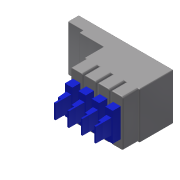
# Autodesk Inventor part: cRio FRC II with 3 modules 2 breakouts
Saved by Autodesk Inventor 2013 (Build 170138000, 138)
## iProperties
Created: 2013-12-22
Part Number: cRio FRC II with 3 modules 2 breakouts
Material: Iron, Cast
Document SubType Name: Modeling
Designer: Nemo
Mass: 1124.91 g
Surface Area: 772.846 cm^2
Volume: 929.109 cm^3
Density: 1.21074 g/cm^3
Author: Nemo
Autodesk Inventor part; units mm, degrees
ref_plane "YZ Plane" through (0, 0, 0) normal (1, 0, 0) x (0, 1, 0)
ref_plane "XZ Plane" through (0, 0, 0) normal (0, 1, 0) x (-1, 0, 0)
ref_plane "XY Plane" through (0, 0, 0) normal (0, 0, 1) x (1, 0, 0)
sketch "Sketch1" plane through (0, 0, 0) normal (0, 0, 1) x (1, 0, 0)
  line L0 (0, 0) -> (179.578, 0)
  line L1 (179.578, 0) -> (179.578, 88.138)
  line L2 (179.578, 88.138) -> (0, 88.138)
  line L3 (0, 88.138) -> (0, 0)
  dimension "d0" = 179.578
  dimension "d1" = 88.138
  constraints: 8 end point, 2 parallel, 1 horizontal, 1 perpendicular
  measures "d0" distance of L2.end L1.end
  measures "d1" distance of L1.end L0.end
extrude "Extrusion1" add sketch "Sketch1" along normal blind 27.94
sketch "Sketch2" plane through (0, 0, 27.94) normal (0, 0, 1) x (1, 0, 0)
  line L0 (0, 0) -> (179.578, 0) projected
  line L1 (179.578, 88.138) -> (75.184, 88.138)
  line L2 (75.184, 88.138) -> (75.184, 0)
  line L3 (75.184, 0) -> (179.578, 0)
  line L4 (179.578, 0) -> (179.578, 88.138)
  dimension "d4" = 104.394
  constraints: 8 end point, 2 parallel, 1 horizontal, 1 perpendicular, 1 point on line
  measures "d4" distance between parallel lines of L4 L2
extrude "Extrusion2" add sketch "Sketch2" along normal blind 36.3474
sketch "Sketch3" plane through (0, 0, 64.2874) normal (0, 0, 1) x (1, 0, 0)
  line L0 (75.184, 0) -> (179.578, 0) projected
  line L1 (179.578, 88.138) -> (75.184, 88.138) projected
  line L2 (75.184, 88.138) -> (75.184, 0) projected
  line L3 (77.724, 88.138) -> (100.584, 88.138)
  line L4 (100.584, 88.138) -> (100.584, 0)
  line L5 (100.584, 0) -> (77.724, 0)
  line L6 (77.724, 0) -> (77.724, 88.138)
  point P0 (0, 0)
  dimension "d8" = 22.86
  dimension "d9" = 2.54
  constraints: 8 end point, 2 parallel, 2 point on line, 1 horizontal, 1 perpendicular
  measures "d8" distance of L4.end L5.end
  measures "d9" distance between parallel lines of L2 L6
extrude "Extrusion3" add sketch "Sketch3" along normal blind 28.6512 contours L6 L1 L4 L0
fillet "Fillet1" radius 3.175 4 edges at (77.724, 0, 78.613) (100.584, 0, 78.613) (77.724, 88.138, 78.613) (100.584, 88.138, 78.613)
pattern_linear "Rectangular Pattern1" count 4 spacing 25.4 along (1, 0, 0) of "Extrusion3", "Fillet1"
sketch "Sketch4" plane through (0, 0, 27.94) normal (0, 0, 1) x (1, 0, 0)
  line L0 (75.184, 88.138) -> (0, 88.138) projected
  line L1 (0, 0) -> (28.956, 0)
  line L2 (28.956, 0) -> (28.956, 88.138)
  line L3 (28.956, 88.138) -> (0, 88.138)
  line L4 (0, 88.138) -> (0, 0)
  dimension "d16" = 28.956
  constraints: 8 end point, 2 parallel, 1 horizontal, 1 perpendicular, 1 point on line
  measures "d16" distance between parallel lines of L4 L2
extrude "Extrusion4" cut sketch "Sketch4" against normal blind 7.4422
fillet "Fillet2" radius 1.5875 64 edges at (28.956, 44.069, 27.94) (52.07, 0, 27.94) (75.184, 44.069, 27.94) (52.07, 88.138, 27.94) (14.478, 0, 20.4978) (0, 0, 10.2489) (89.789, 0, 0) (179.578, 0, 32.1437) (176.5935, 0, 64.2874) (165.354, 0, 92.9386) (152.654, 0, 64.2874) (139.954, 0, 92.9386) (127.254, 0, 64.2874) (114.554, 0, 92.9386) (101.854, 0, 64.2874) (89.154, 0, 92.9386) (78.0415, 0, 64.2874) (75.184, 0, 46.1137) (28.956, 0, 24.2189) (175.8541, 0.9299, 92.9386) (176.784, 44.069, 92.9386) (175.8541, 87.2081, 92.9386) (165.354, 88.138, 92.9386) (154.8539, 87.2081, 92.9386) (153.924, 44.069, 92.9386) (154.8539, 0.9299, 92.9386) (150.4541, 0.9299, 92.9386) (151.384, 44.069, 92.9386) (150.4541, 87.2081, 92.9386) (139.954, 88.138, 92.9386) (129.4539, 87.2081, 92.9386) (128.524, 44.069, 92.9386) (129.4539, 0.9299, 92.9386) (125.0541, 0.9299, 92.9386) (125.984, 44.069, 92.9386) (125.0541, 87.2081, 92.9386) (114.554, 88.138, 92.9386) (104.0539, 87.2081, 92.9386) (103.124, 44.069, 92.9386) (104.0539, 0.9299, 92.9386) (99.6541, 0.9299, 92.9386) (100.584, 44.069, 92.9386) (99.6541, 87.2081, 92.9386) (89.154, 88.138, 92.9386) (78.6539, 87.2081, 92.9386) (77.724, 44.069, 92.9386) (78.6539, 0.9299, 92.9386) (0, 44.069, 20.4978) (0, 88.138, 10.2489) (0, 44.069, 0) (14.478, 88.138, 20.4978) (28.956, 44.069, 20.4978) (75.184, 44.069, 64.2874) (75.184, 88.138, 46.1137) (28.956, 88.138, 24.2189) (78.0415, 88.138, 64.2874) (101.854, 88.138, 64.2874) (127.254, 88.138, 64.2874) (152.654, 88.138, 64.2874) (176.5935, 88.138, 64.2874) (179.578, 88.138, 32.1437) (89.789, 88.138, 0) (179.578, 44.069, 0) (179.578, 44.069, 64.2874)
sketch "Sketch5" plane through (0, 0, 92.9386) normal (0, 0, 1) x (1, 0, 0)
  line L0 (80.899, 86.5505) -> (97.409, 86.5505) construction
  line L1 (79.3115, 3.175) -> (79.3115, 84.963) construction
  line L2 (82.0039, 71.0565) -> (96.3041, 71.0565)
  line L3 (96.3041, 71.0565) -> (96.3041, 17.0815)
  line L4 (96.3041, 17.0815) -> (82.0039, 17.0815)
  line L5 (82.0039, 17.0815) -> (82.0039, 71.0565)
  point P0 (0, 0)
  point P1 (82.0039, 44.069)
  point P2 (79.3115, 44.069)
  point P3 (89.154, 71.0565)
  point P4 (89.154, 86.5505)
  dimension "d21" = 53.975
  dimension "d23" = 14.3002
  constraints: 8 end point, 4 midpoint, 2 parallel, 1 horizontal, 1 horizontal alignment, 1 perpendicular, 1 vertical alignment
  measures "d21" distance of L4.end L2.start
  measures "d23" distance of L2.start L2.end
extrude "Extrusion5" add sketch "Sketch5" along normal blind 15.24 separate body
sketch "Sketch6" plane through (0, 0, 108.1786) normal (0, 0, 1) x (1, 0, 0)
  line L0 (96.3041, 71.0565) -> (82.0039, 71.0565) construction
  line L1 (82.0039, 71.0565) -> (82.0039, 17.0815) construction
  line L2 (84.3915, 58.674) -> (93.9165, 58.674)
  line L3 (93.9165, 58.674) -> (93.9165, 29.464)
  line L4 (93.9165, 29.464) -> (84.3915, 29.464)
  line L5 (84.3915, 29.464) -> (84.3915, 58.674)
  point P0 (0, 0)
  point P1 (84.3915, 44.069)
  point P2 (82.0039, 44.069)
  point P3 (89.154, 58.674)
  point P4 (89.154, 71.0565)
  dimension "d26" = 29.21
  dimension "d28" = 9.525
  constraints: 8 end point, 4 midpoint, 2 parallel, 1 horizontal, 1 horizontal alignment, 1 perpendicular, 1 vertical alignment
  measures "d26" distance of L4.end L2.start
  measures "d28" distance of L2.start L2.end
extrude "Extrusion7" add sketch "Sketch6" along normal blind 15.9766 draft -3 bodies 2
sketch "Sketch7" plane through (0, 0, 124.1552) normal (0, 0, 1) x (1, 0, 0)
  line L0 (93.0792, 30.3013) -> (85.2288, 30.3013) construction
  line L1 (93.0792, 57.8367) -> (90.1882, 57.8367)
  line L2 (90.1882, 57.8367) -> (90.1882, 30.3013)
  line L3 (90.1882, 30.3013) -> (93.0792, 30.3013)
  line L4 (93.0792, 30.3013) -> (93.0792, 57.8367)
  point P0 (0, 0)
  constraints: 8 end point, 2 parallel, 1 horizontal, 1 perpendicular, 1 point on line
extrude "Extrusion8" add sketch "Sketch7" along normal blind 12.7 bodies 2
pattern_linear "Rectangular Pattern2" count 4 spacing 25.4 along (1, 0, 0) of "Extrusion5", "Extrusion7", "Extrusion8" bodies 2
body "Solid1"
body "Solid2"
